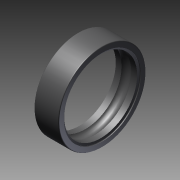
# Autodesk Inventor part: 6002_PART2
Saved by Autodesk Inventor 2016 (Build 200138000, 138)
## iProperties
Category: PARTsolutions
Company: SKF
Created: 2017-09-13
Part Number: 6002_PART2
Catalog Web Link: www.cadenas.de
Description: -Deep groove ball bearings, single row
Vendor: SKF
Document SubType Name: Modeling
Designer: psAdmin
Manufacturer: SKF
Mass: 1.95579 g
Surface Area: 21.9382 cm^2
Volume: 1.95579 cm^3
Density: 1 g/cm^3
Material: Genérico
Appearance: PSOLRGB-175-175-175
PSOL_IDENT_0: {$CADENAS_DATA\23d-libs\skf\bearings_units_and_housings\ball_bearings\deep_groove_ball_bearings\deep
PSOL_IDENT_1: _groove_ball_bearings_single_row\bb1_001_101.prj},190 {VTYP=3D},{NB=6002_PART2},{LINA=6002_PART2},{N
PSOL_IDENT_2: N=BB1_001_101_PART2},{NOPRJ=TRUE},{DATE=14.07.2017 09:01:20},{GEOMDATE=14.07.2017 08:21:21},{VERSION=
PSOL_IDENT_3: },{LINEID=213200},{LINESUBID=-1},{WBVAR=}  {NB=6002_PART2},{LINA=6002_PART2},{KT=DUMMY},{PRODUCTID=1
PSOL_IDENT_4: 050010002},{DESIGNATION=6002},{DD=15.000},{D=32.000},{B=9.000},{HH=-1000000015047466219876688855040.
PSOL_IDENT_5: 000},{DD1=20.500},{DD2=-1000000015047466219876688855040.000},{DD22=-1000000015047466219876688855040.
PSOL_IDENT_6: 000},{D1=26.700},{D2=28.200},{BB=-1000000015047466219876688855040.000},{R12=0.3},{R121=0.300},{R122=
PSOL_IDENT_7: 0.300},{LOAD1=5.850},{LOAD2=2.850},{LOAD3=0.120},{SPEED1=50000},{SPEED2=32000},{MASS=0.030},{PITCH=2
PSOL_IDENT_8: 3.500},{DW=4.762},{Z=9.000},{II=1.000},{TYPEID=105001},{HELP=2.65},{HELP2=1.9},{DD1ALG=10.25},{TAXON
PSOL_IDENT_9: OMY=1},{DESIGN=dgbb1},{MAPPING=BCZ50,DESIGNATION|IRD01,DD|ORD10,D|BCW30,B|ORL64,HH|IRD30,DD1|IRD46,D
PSOL_IDENT_10: D2|IRD43,DD22|ORD30,D1|ORD43,D2|ORL60,BB|ORL03,R121|BCE41,R122|BCC02,LOAD1|BCC16,LOAD2|BCC12,LOAD3|B
PSOL_IDENT_11: CC43,SPEED1|BCC45,SPEED2|BCM01,MASS|BCD50,PITCH|RBD10,DW|BCN81,Z|BCN80,II},{DESIGNLIST=dgbbrs,dgbb1,
PSOL_IDENT_12: dgbb2rs,dgbb2z,dgbbn1,dgbbz},{YALG=10.25000},{HALG=2.75000},{YALG1=13.35000},{HALG1=2.65000},{PITCH1=
PSOL_IDENT_13: 23.50000},{DW1=4.76200},{SH=10.25},{CU=0.8476},{SORT=DD},{PIM=6002}
NT: Deep groove ball bearings, single row
NB: 6002_PART2
NBSYN: $DESIGNATION._PART2
LINA: 6002_PART2
DESIGNATION: 6002
DD: 15.000
D: 32.000
B: 9.000
LOAD1: 5.850
LOAD2: 2.850
LOAD3: 0.120
SPEED1: 50000
SPEED2: 32000
SUPPLIER: SKF
ARTICLENO: 6002_PART2
BOMINFO: 6002_PART2
CREATOR: CADENAS GmbH
Title: 6002_PART2
Author: Cadenas PARTsolutions
Comments: Deep groove ball bearings, single row
Autodesk Inventor part; units mm, degrees
ref_plane "YZ Plane" through (0, 0, 0) normal (1, 0, 0) x (0, 1, 0)
ref_plane "XZ Plane" through (0, 0, 0) normal (0, 1, 0) x (-1, 0, 0)
ref_plane "XY Plane" through (0, 0, 0) normal (0, 0, 1) x (1, 0, 0)
sketch "Sketch_2" plane through (0, 0, 0) normal (0, 0, 1) x (1, 0, 0)
  line L0 (50, 0) -> (-50, 0)
  line L1 (0, 14.1) -> (0.09, 14.1)
  arc A0 (0.45, 14.1) -> (0.09, 14.1) centre (0.27, 14.1) ccw
  line L2 (0.45, 14.1) -> (0.5822, 13.35)
  line L3 (0.5822, 13.35) -> (2.7367, 13.35)
  arc A1 (6.2633, 13.35) -> (2.7367, 13.35) centre (4.5, 11.75) ccw
  line L4 (6.2633, 13.35) -> (8.4178, 13.35)
  line L5 (8.4178, 13.35) -> (8.55, 14.1)
  arc A2 (8.91, 14.1) -> (8.55, 14.1) centre (8.73, 14.1) ccw
  line L6 (8.91, 14.1) -> (9, 14.1)
  line L7 (9, 14.1) -> (9, 15.7)
  arc A3 (9, 15.7) -> (8.7, 16) centre (8.7, 15.7) ccw
  line L8 (8.7, 16) -> (0.3, 16)
  arc A4 (0.3, 16) -> (0, 15.7) centre (0.3, 15.7) ccw
  line L9 (0, 15.7) -> (0, 14.1)
  constraints: 20 end point, 10 point on circle, 5 centre point
revolve "Revolution1" add sketch "Sketch_2" angle 360 about axis through (50, 0, 0) along (1, 0, 0)
body "Solid1"
